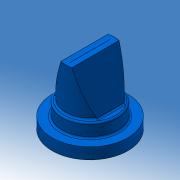
# Autodesk Inventor part: DU039.005-952.01
Saved by Autodesk Inventor 2015 SP1 (Build 190203100, 203)
## iProperties
Created: 2015-02-19
Material: ML952 REZLYN
Vendor: MINIVALVE
Document SubType Name: Modeling
Designer: JORDANJ
Density: 1.2 g/cm^3
Appearance: Rubber (Black)(1)
Project: P-171601
Part Number: DU039.005-952.01
Description: COMPONENT OF AN AUTOMATED LIQUID HANDLING MACHINE SPECIFICALLY DESIGNED FOR THE IN SITU RNA HYBRIDIZATION OF DROSOPHILA EMBRYOS
RuleStatus: InUse
AfterDocSave0: file://Part Number Cleaner
LAB/DEPT: STERN (LAB)
REQUESTING SCIENTIST: STERN, DAVID
SURFACE ROUGHNESS: N/A
DESIGN DEPARTMENT: HHMI: JRC - ID&F
SPECIAL FINISH: N/A
ALTERED ITEM PART NUMBER: N/A
ALTERED ITEM VENDOR: N/A
ALTERED ITEM DESCRIPTION: N/A
Revision Number: 0
Autodesk Inventor part; units mm, degrees
ref_plane "YZ Plane" through (0, 0, 0) normal (1, 0, 0) x (0, 1, 0)
ref_plane "XZ Plane" through (0, 0, 0) normal (0, 1, 0) x (-1, 0, 0)
ref_plane "XY Plane" through (0, 0, 0) normal (0, 0, 1) x (1, 0, 0)
sketch "Sketch1" plane through (0, 0, 0) normal (0, 0, 1) x (1, 0, 0)
  line L0 (0, -1.0008) -> (0, 6.0046) construction
  line L1 (-0.4047, 5.0038) -> (-1.5018, 1.9384)
  line L2 (-1.6213, 1.8542) -> (-1.9177, 1.8542)
  line L3 (-2.0447, 1.7272) -> (-2.0447, 0.9652)
  line L4 (-2.1717, 0.8382) -> (-2.794, 0.8382)
  line L5 (-2.794, 0.8382) -> (-2.794, 0)
  line L6 (-2.794, 0) -> (-1.397, 0)
  line L7 (-1.397, 0) -> (-1.397, 1.6002)
  arc A0 (-1.397, 1.6002) -> (-1.1579, 1.7686) centre (-1.397, 1.8542) ccw
  line L8 (-1.1579, 1.7686) -> (0, 5.0038)
  line L9 (-0.4047, 5.0038) -> (0, 5.0038)
  arc A1 (-1.6213, 1.8542) -> (-1.5018, 1.9384) centre (-1.6213, 1.9812) ccw
  arc A2 (-1.9177, 1.8542) -> (-2.0447, 1.7272) centre (-1.9177, 1.7272) ccw
  arc A3 (-2.1717, 0.8382) -> (-2.0447, 0.9652) centre (-2.1717, 0.9652) ccw
  line L10 (-1.7907, 5.0038) -> (-1.7907, 1.9812)
  arc A4 (-1.9177, 1.8542) -> (-1.7907, 1.9812) centre (-1.9177, 1.9812) ccw
  line L11 (-1.7907, 5.0038) -> (-0.4047, 5.0038)
  point P0 (0, 0)
  dimension "d0" = 5.588
  dimension "d1" = 0.8382
  dimension "d2" = 4.0894
  dimension "d5" = 0.381
  dimension "d7" = 0.127
  dimension "d8" = 5.0038
  dimension "d9" = 1.016
  dimension "d10" = 0.254
  dimension "d11" = 0.254
  dimension "d18" = 2.794
  constraints: 22 end point, 11 point on circle, 9 tangent, 5 centre point, 5 horizontal, 4 vertical, 3 equal radius, 3 point on line, 1 horizontal alignment, 1 parallel
  measures "d0" diameter of L5 L0
  measures "d1" distance of L4.end L5.end
  measures "d2" diameter of L3 L0
  measures "d5" distance between parallel lines of L8 L1
  measures "d7" radius of A1
  measures "d8" distance between parallel lines of L9 L6
  measures "d9" distance between parallel lines of L2 L4
  measures "d10" radius of A0
  measures "d11" distance between parallel lines of L10 L3
  measures "d18" diameter of L7 L0
revolve "Revolution1" add sketch "Sketch1" angle 360 about axis through (0, -10, 0) along (0, 1, 0)
extrude "Extrusion1" cut sketch "Sketch1" along normal through all both and the other way through all contours L1 A1 L2 A4 L10 L11
mirror "Mirror1" about plane through (0, 0, 0) normal (1, 0, 0) of "Extrusion1"
sketch "Sketch2" plane through (-0.4047, 5.0038, 1.7444) normal (0, 1, 0) x (1, 0, 0)
  line L0 (0.4047, 3.2277) -> (0.4047, 0.261) construction
  line L1 (0.4034, 3.2277) -> (0.4059, 3.2277)
  line L2 (0.4059, 3.2277) -> (0.4059, 0.261)
  line L3 (0.4059, 0.261) -> (0.4034, 0.261)
  line L4 (0.4034, 0.261) -> (0.4034, 3.2277)
  point P0 (0.4047, 1.7444)
  dimension "d15" = 0.0025
  constraints: 10 end point, 4 midpoint, 2 parallel, 1 horizontal, 1 perpendicular, 1 vertical
  measures "d15" distance of L1.start L1.end
extrude "Extrusion2" cut sketch "Sketch2" against normal blind 0.0254
body "Solid1"
